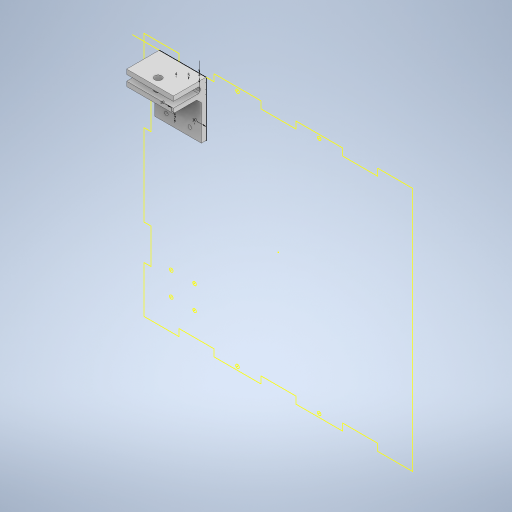
# Autodesk Inventor part: крепеж валика
Saved by Autodesk Inventor 2024.2 (Build 282272000, 272)
## iProperties
Created: 2026-02-03
Part Number: крепеж валика
Material: Типовые
Document SubType Name: Modeling
Designer: Service
Density: 1 g/cm^3
Appearance: По умолчанию
Author: Service
Autodesk Inventor part; units mm, degrees
ref_plane "YZ Plane" through (0, 0, 0) normal (1, 0, 0) x (0, 1, 0)
ref_plane "XZ Plane" through (0, 0, 0) normal (0, 1, 0) x (-1, 0, 0)
ref_plane "XY Plane" through (0, 0, 0) normal (0, 0, 1) x (1, 0, 0)
sketch "Эскиз1" plane through (0, 0, 0) normal (0, 0, 1) x (1, 0, 0)
  line L0 (-76.034, 99) -> (-125.034, 99) projected
  line L1 (-56.034, 99) -> (-73.034, 99) projected
  circle A0 centre (-71.767, -79) radius 1.5 projected
  circle A1 centre (-91.767, -59) radius 1.5 projected
  circle A2 centre (-91.767, -79) radius 1.5 projected
  circle A3 centre (-71.767, -59) radius 1.5 projected
  circle A4 centre (-71.767, 79) radius 1.5 projected
  circle A5 centre (-71.767, 59) radius 1.5 projected
  circle A6 centre (-91.767, 79) radius 1.5 projected
  circle A7 centre (-91.767, 59) radius 1.5 projected
  circle A8 centre (35, -102) radius 1.5 projected
  circle A9 centre (-35, 102) radius 1.5 projected
  circle A10 centre (-35, -102) radius 1.5 projected
  circle A11 centre (35, 102) radius 1.5 projected
  line L2 (15, -105) -> (55, -105) projected
  line L3 (55, -105) -> (55, -99) projected
  line L4 (55, -99) -> (85, -99) projected
  line L5 (85, -99) -> (85, -105) projected
  line L6 (85, -105) -> (115, -105) projected
  line L7 (115, -105) -> (115, 105) projected
  line L8 (115, 105) -> (85, 105) projected
  line L9 (85, 105) -> (85, 99) projected
  line L10 (85, 99) -> (55, 99) projected
  line L11 (55, 99) -> (55, 105) projected
  line L12 (55, 105) -> (15, 105) projected
  line L13 (15, 105) -> (15, 99) projected
  line L14 (15, 99) -> (-15, 99) projected
  line L15 (-15, 99) -> (-15, 105) projected
  line L16 (-15, 105) -> (-55, 105) projected
  line L17 (-55, 105) -> (-55, 99) projected
  line L18 (-55, 99) -> (-85, 99) projected
  line L19 (-85, 99) -> (-85, 105) projected
  line L20 (-85, 105) -> (-115, 105) projected
  line L21 (-115, 105) -> (-115, 65) projected
  line L22 (-115, 65) -> (-109, 65) projected
  line L23 (-109, 65) -> (-109, 35) projected
  line L24 (-109, 35) -> (-115, 35) projected
  line L25 (-115, 35) -> (-115, -35) projected
  line L26 (-115, -35) -> (-109, -35) projected
  line L27 (-109, -35) -> (-109, -65) projected
  line L28 (-109, -65) -> (-115, -65) projected
  line L29 (-115, -65) -> (-115, -105) projected
  line L30 (-115, -105) -> (-85, -105) projected
  line L31 (-85, -105) -> (-85, -99) projected
  line L32 (-85, -99) -> (-55, -99) projected
  line L33 (-55, -99) -> (-55, -105) projected
  line L34 (-55, -105) -> (-15, -105) projected
  line L35 (-15, -105) -> (-15, -99) projected
  line L36 (-15, -99) -> (15, -99) projected
  line L37 (15, -99) -> (15, -105) projected
  line L38 (-61.767, 52) -> (-101.767, 52)
  line L39 (-101.767, 52) -> (-101.767, 99)
  line L40 (-101.767, 99) -> (-61.767, 99)
  line L41 (-61.767, 99) -> (-61.767, 52)
  line L42 (-101.767, 99) -> (-61.767, 99)
  line L43 (-61.767, 99) -> (-61.767, 95)
  line L44 (-61.767, 95) -> (-101.767, 95)
  line L45 (-101.767, 95) -> (-101.767, 99)
  line L46 (-61.767, 90) -> (-101.767, 90)
  line L47 (-101.767, 90) -> (-101.767, 86)
  line L48 (-101.767, 86) -> (-61.767, 86)
  line L49 (-61.767, 86) -> (-61.767, 90)
  point P0 (0, 0)
  dimension "d0" = 10
  dimension "d1" = 10
  dimension "d2" = 7
  dimension "d3" = 4
  dimension "d4" = 5
  dimension "d5" = 4
  constraints: 24 end point, 6 parallel, 3 horizontal, 3 perpendicular, 3 point on line, 1 collinear
  measures "d0" distance from line of A5.centre L41
  measures "d1" distance from line of L39 A7.centre
  measures "d2" distance from line of L38 A7.centre
  measures "d3" distance between parallel lines of L42 L44
  measures "d4" distance between parallel lines of L44 L46
  measures "d5" distance between parallel lines of L46 L48
extrude "Выдавливание1" add sketch "Эскиз1" along normal blind 4 contours L18 L1 L41 L44 L39 L0 | L44 L41 L46 L39 | L46 L41 L48 L39 | L48 L41 L38 L39
extrude "Выдавливание2" add sketch "Эскиз1" along normal blind 28 contours L18 L1 L41 L44 L39 L0 | L46 L41 L48 L39
chamfer "Фаска1" distance 4 angle 45 1 edges at (-81.767, 86, 4)
chamfer "Фаска2" distance 2.5 angle 45 2 edges at (-81.767, 95, 4) (-81.767, 90, 4)
fillet "Сопряжение1" radius 2 4 edges at (-61.767, 92.5, 4) (-81.767, 92.4999, 4) (-101.767, 92.5, 4) (-81.767, 92.5001, 4)
sketch "Эскиз2" plane through (-101.767, 86, 28) normal (0, -1, 0) x (1, 0, 0)
  circle A0 centre (20, -7) radius 3
  line L0 (0, -28) -> (40, -28) projected
  line L1 (0, -20) -> (0, 0) projected
  point P0 (101.767, -28)
  dimension "d17" = 6
  dimension "d18" = 21
  dimension "d19" = 20
  constraints: 1 centre point
  measures "d17" diameter of A0
  measures "d18" distance from line of L0 A0.centre
  measures "d19" distance from line of L1 A0.centre
extrude "Выдавливание3" cut sketch "Эскиз2" against normal blind 24.75
